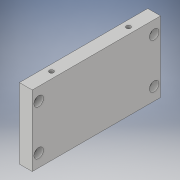
# Autodesk Inventor part: BatteryFrontPlate
Saved by Autodesk Inventor 2019 (Build 230136000, 136)
## iProperties
Created: 2018-11-18
Part Number: BatteryFrontPlate
Material: Generic
Document SubType Name: Modeling
Designer: james
Density: 1 g/cm^3
Appearance: Default
Author: james
Autodesk Inventor part; units mm, degrees
ref_plane "YZ Plane" through (0, 0, 0) normal (1, 0, 0) x (0, 1, 0)
ref_plane "XZ Plane" through (0, 0, 0) normal (0, 1, 0) x (-1, 0, 0)
ref_plane "XY Plane" through (0, 0, 0) normal (0, 0, 1) x (1, 0, 0)
sketch "Sketch1" plane through (0, 0, 0) normal (0, 1, 0) x (-1, 0, 0)
  line L0 (6.7628, 14.9608) -> (-5.9372, 14.9608)
  line L1 (-5.9372, 14.9608) -> (-5.9372, -112.0392)
  line L2 (-5.9372, -112.0392) -> (6.7628, -112.0392)
  line L3 (6.7628, -112.0392) -> (6.7628, 14.9608)
  point P0 (0, 0)
  dimension "d0" = 12.7
  dimension "d1" = 127
  constraints: 8 end point, 2 parallel, 1 horizontal, 1 perpendicular
  measures "d0" distance of L0.start L0.end
  measures "d1" distance of L2.end L0.start
extrude "Extrusion1" add sketch "Sketch1" along normal blind 69.85
sketch "Sketch2" plane through (0, 69.85, 0) normal (0, 1, 0) x (1, 0, 0)
  line L0 (5.9372, 112.0392) -> (-6.7628, 112.0392) projected
  line L1 (5.9372, -14.9608) -> (5.9372, 112.0392) projected
  line L2 (-6.7628, -14.9608) -> (5.9372, -14.9608) projected
  point P0 (0, 0)
  point P1 (-0.4128, 10.4392)
  point P2 (-0.4128, 86.6392)
  dimension "d4" = 25.4
  dimension "d5" = 6.35
  dimension "d6" = 25.4
  dimension "d7" = 6.35
  measures "d4" distance from line of point (-0.413, 86.639) L0
  measures "d5" distance from line of L1 point (-0.413, 86.639)
  measures "d6" distance from line of L2 point (-0.413, 10.439)
  measures "d7" distance from line of L1 point (-0.413, 10.439)
hole "Hole1" at (-0.4128, 69.85, -10.4392) at (-0.4128, 69.85, -86.6392) direction (0, -1, 0) diameter 4.318 end through all
sketch "Sketch3" plane through (5.9372, 0, 14.9608) normal (1, 0, 0) x (0, 0, -1)
  line L0 (0, 0) -> (0, 69.85) projected
  line L1 (0, 0) -> (127, 0) projected
  line L2 (0, 69.85) -> (127, 69.85) projected
  line L3 (127, 0) -> (127, 69.85) projected
  point P0 (14.9608, 0)
  point P1 (6.35, 57.15)
  point P2 (6.35, 12.7)
  point P3 (120.65, 57.15)
  point P4 (120.65, 12.7)
  dimension "d15" = 6.35
  dimension "d16" = 6.35
  dimension "d17" = 12.7
  dimension "d18" = 12.7
  dimension "d19" = 12.7
  dimension "d20" = 6.35
  dimension "d21" = 6.35
  dimension "d22" = 12.7
  measures "d15" distance from line of L0 point (6.35, 57.15)
  measures "d16" distance from line of L0 point (6.35, 12.7)
  measures "d17" distance from line of L1 point (6.35, 12.7)
  measures "d18" distance from line of L2 point (6.35, 57.15)
  measures "d19" distance from line of L1 point (120.65, 12.7)
  measures "d20" distance from line of L3 point (120.65, 12.7)
  measures "d21" distance from line of L3 point (120.65, 57.15)
  measures "d22" distance from line of L2 point (120.65, 57.15)
hole "Hole2" at (5.9372, 57.15, 8.6108) at (5.9372, 12.7, 8.6108) at (5.9372, 57.15, -105.6892) at (5.9372, 12.7, -105.6892) direction (-1, 0, 0) diameter 4.064 end through all counterbore diameter 9.525 counterbore depth 6.35
body "Solid1"
